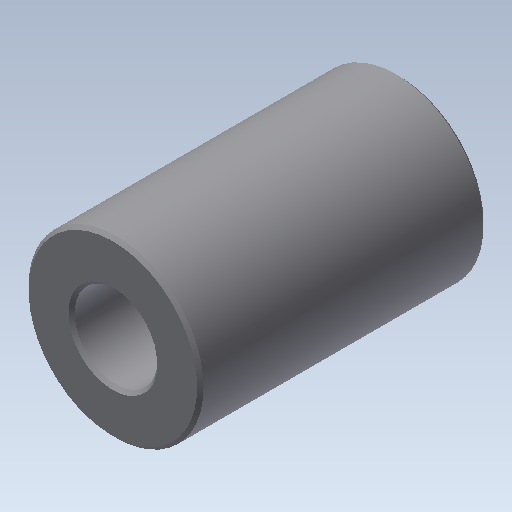
# Autodesk Inventor part: wheel_tube
Saved by Autodesk Inventor 2020.3 (Build 243373000, 373)
## iProperties
Created: 2015-11-09
Part Number: wheel_tube
Material: Ogólny
Document SubType Name: Modeling
Designer: Marcin
Density: 1 g/cm^3
Appearance: Domyślna
Mass: 1.35459 g
Surface Area: 10.4688 cm^2
Volume: 1.35459 cm^3
Author: Marcin
Autodesk Inventor part; units mm, degrees
ref_plane "YZ Plane" through (0, 0, 0) normal (1, 0, 0) x (0, 1, 0)
ref_plane "XZ Plane" through (0, 0, 0) normal (0, 1, 0) x (-1, 0, 0)
ref_plane "XY Plane" through (0, 0, 0) normal (0, 0, 1) x (1, 0, 0)
sketch "Szkic1" plane through (0, 0, 0) normal (0, 0, 1) x (1, 0, 0)
  circle A0 centre (0, 0) radius 5.5
  dimension "d0" = 11
  constraints: 1 centre point, 1 coincident
  measures "d0" diameter of A0
extrude "Wyciągnięcie proste1" add sketch "Szkic1" along normal blind 18
sketch "Szkic2" plane through (0, 0, 18) normal (0, 0, 1) x (1, 0, 0)
  circle A0 centre (0, 0) radius 2.6
  dimension "d3" = 5.2
  constraints: 1 centre point, 1 coincident
  measures "d3" diameter of A0
extrude "Wyciągnięcie proste2" cut sketch "Szkic2" against normal blind 9
sketch "Szkic3" plane through (0, 0, 0) normal (0, 0, -1) x (-1, 0, 0)
  circle A0 centre (0, 0) radius 2.4
  dimension "d6" = 4.8
  constraints: 1 centre point, 1 coincident
  measures "d6" diameter of A0
extrude "Wyciągnięcie proste3" cut sketch "Szkic3" against normal blind 9
chamfer "Faza1" distance 0.2 angle 45 4 edges at (-5.5, 0, 18) (-5.5, 0, 0) (2.4, 0, 0) (-2.6, 0, 18)
